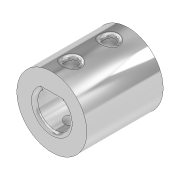
# Autodesk Inventor part: 5mm Coupler
Saved by Autodesk Inventor 2020 (Build 240168000, 168)
## iProperties
Created: 2021-06-28
Part Number: 5mm Coupler
Material: Generic
Document SubType Name: Modeling
Designer: Coy
Density: 1 g/cm^3
Appearance: Chrome - Polished
Author: Coy
Autodesk Inventor part; units mm, degrees
ref_plane "YZ Plane" through (0, 0, 0) normal (1, 0, 0) x (0, 1, 0)
ref_plane "XZ Plane" through (0, 0, 0) normal (0, 1, 0) x (-1, 0, 0)
ref_plane "XY Plane" through (0, 0, 0) normal (0, 0, 1) x (1, 0, 0)
sketch "Sketch1" plane through (0, 0, 0) normal (0, 0, 1) x (1, 0, 0)
  arc A0 (-1.5, 2) -> (1.5, 2) centre (0, 0) ccw construction
  circle A1 centre (0, 0) radius 4
  circle A2 centre (0, 0) radius 5.5
  arc A3 (-1.5, 2) -> (1.5, 2) centre (0, 0) ccw construction
  line L0 (-1.5, 2) -> (1.5, 2) construction
  arc A4 (-1.62, 2.16) -> (1.62, 2.16) centre (0, 0) ccw
  line L1 (1.62, 2.16) -> (-1.62, 2.16)
  dimension "d0" = 5
  dimension "d1" = 8
  dimension "d17" = 3
  dimension "d18" = 5
  dimension "d19" = 2
  dimension "d20" = 0.2
  constraints: 6 point on circle, 5 centre point, 4 end point, 3 coincident, 1 horizontal, 1 parallel
  measures "d0" diameter of A0
  measures "d1" diameter of A1
  measures "d17" radial gap between concentric circles of A0 A2
  measures "d18" diameter of A3
  measures "d19" distance from line of point (0, 0) L0
  measures "d20" radial gap between concentric circles of A0 A4
extrude "Extrusion1" add sketch "Sketch1" along normal blind 12 contours A1 | A2
sketch "Sketch3" plane through (-1.62, 2.16, 0) normal (0, -1, 0) x (1, 0, 0)
  line L0 (0, 0) -> (3.24, 0) projected
  line L1 (3.24, 0) -> (3.24, 12) projected
  line L2 (0, 12) -> (3.24, 12) projected
  line L3 (0, 0) -> (0, 12) projected
  line L4 (3.24, 0) -> (3.24, 12) construction
  line L5 (3.24, 6) -> (3.24, 0) construction
  line L6 (0, 12) -> (3.24, 12) construction
  line L7 (3.24, 6) -> (3.24, 12) construction
  line L8 (3.24, 3) -> (0, 3) construction
  line L9 (0, 0) -> (0, 12) construction
  line L10 (3.24, 9) -> (0, 9) construction
  circle A0 centre (1.62, 3) radius 0.95
  circle A1 centre (1.62, 9) radius 0.95
  point P0 (1.62, 0)
  dimension "d21" = 1.9
  dimension "d22" = 1.9
  constraints: 8 end point, 5 midpoint, 2 centre point, 2 point on line, 1 collinear, 1 horizontal, 1 perpendicular, 1 vertical
  measures "d21" diameter of A0
  measures "d22" diameter of A1
extrude "Extrusion3" cut sketch "Sketch3" along normal through all both and the other way through all contours A0 | A1
fillet "Fillet2" radius 0.5 8 edges at (0, 2.16, 12) (0, -2.7, 12) (0, 2.16, 0) (0, -2.7, 0) (-0.9487, 5.4176, 3.0506) (-0.9487, 5.4176, 9.0506) (-0.9487, -5.4176, 3.0506) (-0.9487, -5.4176, 9.0506)
body "Solid1"
